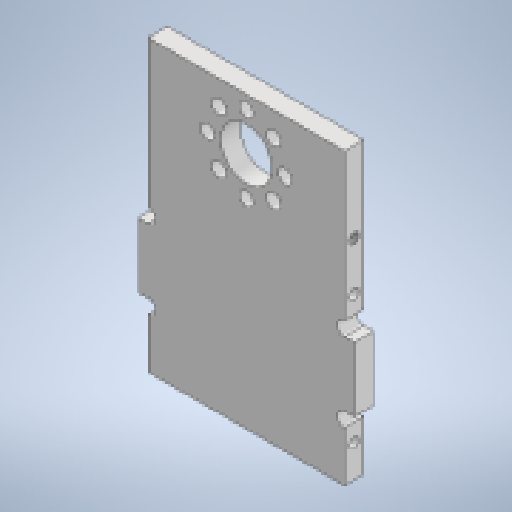
# Autodesk Inventor part: kosiyo
Saved by Autodesk Inventor 2025.1 (Build 291241000, 241)
## iProperties
Created: 2024-08-31
Part Number: kosiyo
Material: 一般
Document SubType Name: Modeling
Designer: right
Density: 1 g/cm^3
Appearance: 既定
Author: right
Autodesk Inventor part; units mm, degrees
ref_plane "YZ Plane" through (0, 0, 0) normal (1, 0, 0) x (0, 1, 0)
ref_plane "XZ Plane" through (0, 0, 0) normal (0, 1, 0) x (-1, 0, 0)
ref_plane "XY Plane" through (0, 0, 0) normal (0, 0, 1) x (1, 0, 0)
sketch "スケッチ1" plane through (0, 0, 0) normal (0, 0, 1) x (1, 0, 0)
  line L0 (-15.25, -22.5) -> (15.25, -22.5)
  line L1 (15.25, -22.5) -> (15.25, 22.5)
  line L2 (15.25, 22.5) -> (-15.25, 22.5)
  line L3 (-15.25, 22.5) -> (-15.25, -22.5)
  line L4 (-15.25, -22.5) -> (15.25, 22.5) construction
  line L5 (15.25, -22.5) -> (-15.25, 22.5) construction
  point P0 (0, 0)
  dimension "d0" = 30.5
  dimension "d1" = 45
  constraints: 12 end point, 2 midpoint, 2 parallel, 1 horizontal, 1 perpendicular
  measures "d0" distance of L2.end L1.end
  measures "d1" distance of L2.end L0.start
extrude "押し出し1" add sketch "スケッチ1" along normal blind 3
sketch "スケッチ2" plane through (0, 0, 3) normal (0, 0, 1) x (1, 0, 0)
  line L0 (-15.25, -2.5) -> (-16.75, -2.5)
  line L1 (-16.75, -2.5) -> (-16.75, -12.5)
  line L2 (-16.75, -12.5) -> (-15.25, -12.5)
  line L3 (-15.25, -12.5) -> (-15.25, -2.5)
  line L4 (-15.25, 22.5) -> (-15.25, -22.5) projected
  line L5 (-15.25, -22.5) -> (15.25, -22.5) projected
  circle A0 centre (-15.25, -13.6) radius 1.1
  circle A1 centre (-15.25, -1.4) radius 1.1
  line L6 (15.25, 22.5) -> (-15.25, 22.5) construction
  line L7 (0, 22.5) -> (0, 0) construction
  line L8 (15.25, -2.5) -> (16.75, -2.5)
  line L9 (16.75, -2.5) -> (16.75, -12.5)
  line L10 (16.75, -12.5) -> (15.25, -12.5)
  line L11 (15.25, -12.5) -> (15.25, -2.5)
  circle A2 centre (15.25, -13.6) radius 1.1
  circle A3 centre (15.25, -1.4) radius 1.1
  point P0 (-15.25, -0.3)
  point P1 (-15.25, -14.7)
  dimension "d7" = 2.2
  dimension "d4" = 10
  dimension "d5" = 1.5
  dimension "d6" = 10
  constraints: 18 end point, 6 symmetric about line, 3 point on line, 3 vertical, 2 parallel, 2 vertical alignment, 1 horizontal, 1 midpoint, 1 perpendicular, 10 other
  measures "d4" distance of L0.end L1.end
  measures "d5" distance of L0.start L0.end
  measures "d6" distance between parallel lines of L5 L2
extrude "押し出し2" add sketch "スケッチ2" against normal up to surface (3 mm away) contours L3 L2 L1 L0 | L8 L9 L10 L11
extrude "押し出し3" cut sketch "スケッチ2" against normal through all contours A0 L4 | L4 A1 | A2 | A3 picked at (-14.7226, -13.8557) picked at (-14.9196, -1.2409)
sketch "スケッチ3" plane through (-15.25, 22.5, 0) normal (-1, 0, 0) x (0, 0, 1)
  line L0 (3, -25) -> (0, -25) projected
  line L1 (3, -35) -> (0, -35) projected
  point P0 (0, -22.5)
  point P1 (1.5, -20)
  point P2 (1.5, -40)
  point P3 (1.5, -25)
  point P4 (1.5, -35)
  point P5 (1.5, -25)
  point P6 (1.5, -35)
  dimension "d12" = 5
  dimension "d13" = 5
  constraints: 4 midpoint, 2 vertical alignment
  measures "d12" distance of point (1.5, -25) point (1.5, -20)
  measures "d13" distance of point (1.5, -35) point (1.5, -40)
hole "穴1" at (-15.25, 2.5, 1.5) at (-15.25, -17.5, 1.5) direction (1, 0, 0) diameter 1.567 end through all thread size "M2x0.4" class "6H" standard "ISO Metric profile"
sketch "スケッチ4" plane through (0, 0, 3) normal (0, 0, 1) x (1, 0, 0)
  circle A0 centre (0, 14.5) radius 8
  line L0 (15.25, 22.5) -> (-15.25, 22.5) projected
  circle A1 centre (0, 14.5) radius 4
  circle A2 centre (0, 14.5) radius 6 construction
  circle A3 centre (0, 8.5) radius 1.1
  circle A4 centre (4.2426, 10.2574) radius 1.1
  circle A5 centre (6, 14.5) radius 1.1
  circle A6 centre (4.2426, 18.7426) radius 1.1
  circle A7 centre (0, 20.5) radius 1.1
  circle A8 centre (-4.2426, 18.7426) radius 1.1
  circle A9 centre (-6, 14.5) radius 1.1
  circle A10 centre (-4.2426, 10.2574) radius 1.1
  point P0 (0, 0)
  point P1 (0, 22.5)
  dimension "d23" = 12
  dimension "d21" = 16
  dimension "d22" = 8
  dimension "d24" = 2.2
  dimension "d27" = 360
  constraints: 10 centre point, 3 vertical alignment, 2 coincident, 1 midpoint, 1 tangent, 19 other
  measures "d21" diameter of A0
  measures "d22" diameter of A1
  measures "d24" diameter of A3
extrude "押し出し4" cut sketch "スケッチ4" against normal through all contours A1 | A3 | A4 | A5 | A6 | A7 | A8 | A9 | A10
equation "\"d13\" = d12"
